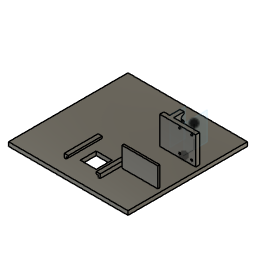
tapa mecatronica v7 (Autodesk Fusion 360 design; units mm, degrees)
Autodesk Fusion 360 part; units mm, degrees
sketch "Boceto1" plane through (0, 0, 0) normal (0, 0, 1) x (1, 0, 0)
  line L0 (-150, -150) -> (150, -150)
  line L1 (150, -150) -> (150, 150)
  line L2 (150, 150) -> (-150, 150)
  line L3 (-150, 150) -> (-150, -150)
  dimension "d1" = 300
  dimension "d2" = 300
  constraint horizontal L0
  constraint vertical L1
  constraint horizontal L2
  constraint vertical L3
  measures "d1" distance of L0.start L0.end
  measures "d2" distance of L0.start L2.end
extrude "Extruir1" add sketch "Boceto1" along normal blind 10
sketch "Boceto2" plane through (0, 0, 10) normal (0, 0, 1) x (-1, 0, 0)
  line L0 (150, -150) -> (150, 150)
  line L1 (150, 150) -> (-150, 150)
  line L2 (-150, 150) -> (-150, -150)
  line L3 (-150, -150) -> (150, -150)
  line L4 (20, 100) -> (-20, 100)
  line L5 (-20, 100) -> (-20, 60)
  line L6 (-20, 60) -> (20, 60)
  line L7 (20, 60) -> (20, 100)
  dimension "d5" = 40
  dimension "d6" = 40
  constraint horizontal L4
  constraint vertical L5
  constraint horizontal L6
  constraint vertical L7
  measures "d5" distance of L5.end L6.end
  measures "d6" distance of L4.start L6.end
shell "Vaciado1" thickness 10 removed faces 1 at (-50, 50, 10)
extrude "Extruir2" cut sketch "Boceto2" against normal blind 10 contours L4 L5 L6 L7
sketch "Boceto3" plane through (0, 0, 10) normal (0, 0, 1) x (-1, 0, 0)
  line L0 (-20, 100) -> (20, 100)
  line L1 (20, 100) -> (20, 60)
  line L2 (20, 60) -> (-20, 60)
  line L3 (-20, 60) -> (-20, 100)
  line L4 (150, -150) -> (150, 150)
  line L5 (150, 150) -> (-150, 150)
  line L6 (-150, 150) -> (-150, -150)
  line L7 (-150, -150) -> (150, -150)
  line L8 (-50, 60) -> (-140, 60)
  line L9 (-140, 60) -> (-140, 65)
  line L10 (-140, 65) -> (-50, 65)
  line L11 (-50, 65) -> (-50, 60)
  constraint horizontal L8
  constraint vertical L9
  constraint horizontal L10
  constraint vertical L11
extrude "Extruir3" add sketch "Boceto3" along normal blind 50 contours L8 L9 L10 L11
sketch "Boceto4" plane through (0, 0, 10) normal (0, 0, 1) x (-1, 0, 0)
  line L0 (-50, 65) -> (-50, 60)
  line L1 (-50, 60) -> (-140, 60)
  line L2 (-140, 60) -> (-140, 65)
  line L3 (-140, 65) -> (-50, 65)
  line L4 (-20, 100) -> (20, 100)
  line L5 (20, 100) -> (20, 60)
  line L6 (20, 60) -> (-20, 60)
  line L7 (-20, 60) -> (-20, 100)
  line L8 (150, -150) -> (150, 150)
  line L9 (150, 150) -> (-150, 150)
  line L10 (-150, 150) -> (-150, -150)
  line L11 (-150, -150) -> (150, -150)
  line L12 (45, 30) -> (40, 30)
  line L13 (40, 30) -> (40, 115)
  line L14 (40, 115) -> (45, 115)
  line L15 (45, 115) -> (45, 30)
  line L16 (35, 30) -> (30, 30)
  line L17 (30, 30) -> (30, 115)
  line L18 (30, 115) -> (35, 115)
  line L19 (35, 115) -> (35, 30)
  line L20 (-30, 30) -> (-35, 30)
  line L21 (-35, 30) -> (-35, 115)
  line L22 (-35, 115) -> (-30, 115)
  line L23 (-30, 115) -> (-30, 30)
  line L24 (-40, 30) -> (-45, 30)
  line L25 (-45, 30) -> (-45, 115)
  line L26 (-45, 115) -> (-40, 115)
  line L27 (-40, 115) -> (-40, 30)
  constraint horizontal L12
  constraint vertical L13
  constraint horizontal L14
  constraint vertical L15
  constraint horizontal L16
  constraint vertical L17
  constraint horizontal L18
  constraint vertical L19
  constraint horizontal L20
  constraint vertical L21
  constraint horizontal L22
  constraint vertical L23
  constraint horizontal L24
  constraint vertical L25
  constraint horizontal L26
  constraint vertical L27
extrude "Extruir4" add sketch "Boceto4" along normal blind 10 contours L12 L13 L14 L15 | L16 L17 L18 L19 | L20 L21 L22 L23 | L24 L25 L26 L27
sketch "Boceto5" plane through (-40, 0, 0) normal (1, 0, 0) x (0, 1, 0)
  line L0 (-115, 10) -> (-30, 10)
  line L1 (-30, 10) -> (-30, 20)
  line L2 (-30, 20) -> (-115, 20)
  line L3 (-115, 20) -> (-115, 10)
  line L4 (-30, 20) -> (-115, 20)
  line L5 (-115, 20) -> (-115, 15)
  line L6 (-115, 15) -> (-30, 15)
  line L7 (-30, 15) -> (-30, 20)
  constraint horizontal L4
  constraint vertical L5
  constraint horizontal L6
  constraint vertical L7
  constraint midpoint L3 L5.end
  constraint coincident L1.end L2.start
extrude "Extruir5" add sketch "Boceto5" along normal blind 5 contours L1 L2 L3 L4 L5 L6 L7
sketch "Boceto6" plane through (35, 0, 0) normal (1, 0, 0) x (0, 1, 0)
  line L0 (-115, 10) -> (-30, 10)
  line L1 (-30, 10) -> (-30, 20)
  line L2 (-30, 20) -> (-115, 20)
  line L3 (-115, 20) -> (-115, 10)
  line L4 (-30, 20) -> (-115, 20)
  line L5 (-115, 20) -> (-115, 15)
  line L6 (-115, 15) -> (-30, 15)
  line L7 (-30, 15) -> (-30, 20)
  constraint horizontal L4
  constraint vertical L5
  constraint horizontal L6
  constraint vertical L7
  constraint midpoint L3 L5.end
  constraint coincident L1.end L2.start
extrude "Extruir6" add sketch "Boceto6" along normal blind 5 contours L1 L2 L3 L4 L5 L6 L7
sketch "Boceto7" plane through (0, 0, 20) normal (0, 0, 1) x (-1, 0, 0)
  line L0 (-30, 115) -> (-45, 115)
  line L1 (-45, 115) -> (-45, 30)
  line L2 (-45, 30) -> (-30, 30)
  line L3 (-30, 30) -> (-30, 115)
  line L4 (-30, 30) -> (-35, 30)
  line L5 (-35, 30) -> (-35, 115)
  line L6 (-35, 115) -> (-30, 115)
  line L7 (-30, 115) -> (-30, 30)
  constraint horizontal L4
  constraint vertical L5
  constraint horizontal L6
  constraint vertical L7
  constraint coincident L0 L5.end
  constraint coincident L2.end L3.start
extrude "Extruir7" cut sketch "Boceto7" against normal blind 10 contours L0 L2 L3 L4 L5 L6 L7
sketch "Boceto8" plane through (0, 0, 20) normal (0, 0, 1) x (-1, 0, 0)
  line L0 (45, 115) -> (30, 115)
  line L1 (30, 115) -> (30, 30)
  line L2 (30, 30) -> (45, 30)
  line L3 (45, 30) -> (45, 115)
  line L4 (30, 30) -> (35, 30)
  line L5 (35, 30) -> (35, 115)
  line L6 (35, 115) -> (30, 115)
  line L7 (30, 115) -> (30, 30)
  constraint horizontal L4
  constraint vertical L5
  constraint horizontal L6
  constraint vertical L7
  constraint coincident L0 L5.end
  constraint coincident L1.end L2.start
extrude "Extruir8" cut sketch "Boceto8" against normal blind 10 contours L0 L1 L2 L4 L5 L6 L7
sketch "Boceto9" plane through (0, 0, 10) normal (0, 0, 1) x (-1, 0, 0)
  line L0 (-40, 115) -> (-40, 30)
  line L1 (-40, 30) -> (-45, 30)
  line L2 (-45, 30) -> (-45, 115)
  line L3 (-45, 115) -> (-40, 115)
  line L4 (45, 115) -> (45, 30)
  line L5 (45, 30) -> (40, 30)
  line L6 (40, 30) -> (40, 115)
  line L7 (40, 115) -> (45, 115)
  line L8 (-50, 65) -> (-50, 60)
  line L9 (-50, 60) -> (-140, 60)
  line L10 (-140, 60) -> (-140, 65)
  line L11 (-140, 65) -> (-50, 65)
  line L12 (-20, 100) -> (20, 100)
  line L13 (20, 100) -> (20, 60)
  line L14 (20, 60) -> (-20, 60)
  line L15 (-20, 60) -> (-20, 100)
  line L16 (150, -150) -> (150, 150)
  line L17 (150, 150) -> (-150, 150)
  line L18 (-150, 150) -> (-150, -150)
  line L19 (-150, -150) -> (150, -150)
  line L20 (-53.6432, 60) -> (-53.6432, -53) construction
  line L21 (-50, -30) -> (-140, -30)
  line L22 (-140, -30) -> (-140, -40)
  line L23 (-140, -40) -> (-50, -40)
  line L24 (-50, -40) -> (-50, -30)
  dimension "d22" = 113
  constraint coincident L9 L20.start
  constraint perpendicular L9 L20
  constraint horizontal L21
  constraint vertical L22
  constraint horizontal L23
  constraint vertical L24
  measures "d22" distance of L20.start L20.end
extrude "Extruir9" add sketch "Boceto9" along normal blind 70 contours L21 L22 L23 L24
sketch "Boceto10" plane through (0, 0, 10) normal (0, 0, 1) x (-1, 0, 0)
  line L0 (-50, -40) -> (-140, -40)
  line L1 (-140, -40) -> (-140, -30)
  line L2 (-140, -30) -> (-50, -30)
  line L3 (-50, -30) -> (-50, -40)
  line L4 (-40, 115) -> (-40, 30)
  line L5 (-40, 30) -> (-45, 30)
  line L6 (-45, 30) -> (-45, 115)
  line L7 (-45, 115) -> (-40, 115)
  line L8 (45, 115) -> (45, 30)
  line L9 (45, 30) -> (40, 30)
  line L10 (40, 30) -> (40, 115)
  line L11 (40, 115) -> (45, 115)
  line L12 (-50, 65) -> (-50, 60)
  line L13 (-50, 60) -> (-140, 60)
  line L14 (-140, 60) -> (-140, 65)
  line L15 (-140, 65) -> (-50, 65)
  line L16 (-20, 100) -> (20, 100)
  line L17 (20, 100) -> (20, 60)
  line L18 (20, 60) -> (-20, 60)
  line L19 (-20, 60) -> (-20, 100)
  line L20 (150, -150) -> (150, 150)
  line L21 (150, 150) -> (-150, 150)
  line L22 (-150, 150) -> (-150, -150)
  line L23 (-150, -150) -> (150, -150)
  line L24 (-100, -40) -> (-133.3526, -40)
  line L25 (-133.3526, -40) -> (-133.3526, -99.3533)
  line L26 (-133.3526, -99.3533) -> (-100, -99.3533)
  line L27 (-100, -99.3533) -> (-100, -40)
  constraint horizontal L24
  constraint vertical L25
  constraint horizontal L26
  constraint vertical L27
  constraint coincident L0 L24.start
extrude "Extruir10" add sketch "Boceto10" along normal blind 70 contours L0 L24 L25 L26 L27
sketch "Boceto11" plane through (100, 0, 0) normal (-1, 0, 0) x (0, -1, 0)
  line L0 (-99.3533, 10) -> (-40, 10)
  line L1 (-40, 10) -> (-40, 80)
  line L2 (-40, 80) -> (-99.3533, 80)
  line L3 (-99.3533, 80) -> (-99.3533, 10)
  line L4 (-40, 10) -> (-65.989, 10) construction
  line L5 (-65.989, 10) -> (-65.989, 67.376) construction
  dimension "d27" = 25.989
  dimension "d28" = 57.376
  constraint coincident L0.end L1.start
  constraint perpendicular L1 L4
  constraint perpendicular L0 L5
  measures "d27" distance of L0.end L4.end
  measures "d28" distance of L4.end L5.end
sketch "Boceto12" plane through (100, 0, 0) normal (-1, 0, 0) x (0, -1, 0)
  circle A0 centre (-66.0255, 67.4058) radius 7.5
  dimension "d30" = 15
  measures "d30" diameter of A0
extrude "Extruir11" cut sketch "Boceto12" against normal blind 10
sketch "Boceto13" plane through (100, 0, 0) normal (-1, 0, 0) x (0, -1, 0)
sketch "Boceto14" plane through (0, 0, 10) normal (0, 0, 1) x (-1, 0, 0)
  line L0 (150, -150) -> (150, 150)
  line L1 (150, 150) -> (-150, 150)
  line L2 (-150, 150) -> (-150, -150)
  line L3 (-150, -150) -> (150, -150)
  line L4 (-20, 100) -> (20, 100)
  line L5 (20, 100) -> (20, 60)
  line L6 (20, 60) -> (-20, 60)
  line L7 (-20, 60) -> (-20, 100)
  line L8 (-50, 65) -> (-50, 60)
  line L9 (-50, 60) -> (-140, 60)
  line L10 (-140, 60) -> (-140, 65)
  line L11 (-140, 65) -> (-50, 65)
  line L12 (45, 115) -> (45, 30)
  line L13 (45, 30) -> (40, 30)
  line L14 (40, 30) -> (40, 115)
  line L15 (40, 115) -> (45, 115)
  line L16 (-40, 115) -> (-40, 30)
  line L17 (-40, 30) -> (-45, 30)
  line L18 (-45, 30) -> (-45, 115)
  line L19 (-45, 115) -> (-40, 115)
  line L20 (-100, -40) -> (-100, -99.3533)
  line L21 (-100, -99.3533) -> (-133.3526, -99.3533)
  line L22 (-133.3526, -99.3533) -> (-133.3526, -40)
  line L23 (-133.3526, -40) -> (-140, -40)
  line L24 (-140, -40) -> (-140, -30)
  line L25 (-140, -30) -> (-50, -30)
  line L26 (-50, -30) -> (-50, -40)
  line L27 (-50, -40) -> (-100, -40)
  line L28 (-65, -40) -> (-75, -40)
  line L29 (-75, -40) -> (-75, -79)
  line L30 (-75, -79) -> (-65, -79)
  line L31 (-65, -79) -> (-65, -40)
  constraint horizontal L28
  constraint vertical L29
  constraint horizontal L30
  constraint vertical L31
  constraint coincident L27 L28.start
extrude "Extruir12" add sketch "Boceto14" along normal blind 70 contours L27 L28 L29 L30 L31
sketch "Boceto15" plane through (100, 0, 0) normal (-1, 0, 0) x (0, -1, 0)
  circle A0 centre (-66, 67.4) radius 7.5
  dimension "d35" = 15
  measures "d35" diameter of A0
extrude "Extruir13" cut sketch "Boceto15" along normal blind 100
sketch "Boceto16" plane through (0, 0, 80) normal (0, 0, 1) x (-1, 0, 0)
  line L0 (-50, -40) -> (-50, -30)
  line L1 (-50, -30) -> (-140, -30)
  line L2 (-140, -30) -> (-140, -40)
  line L3 (-140, -40) -> (-133.3526, -40)
  line L4 (-133.3526, -40) -> (-133.3526, -99.3533)
  line L5 (-133.3526, -99.3533) -> (-100, -99.3533)
  line L6 (-100, -99.3533) -> (-100, -40)
  line L7 (-100, -40) -> (-75, -40)
  line L8 (-75, -40) -> (-75, -79)
  line L9 (-75, -79) -> (-65, -79)
  line L10 (-65, -79) -> (-65, -40)
  line L11 (-65, -40) -> (-50, -40)
  line L12 (-100, -99.3533) -> (-133.3526, -99.3533)
  line L13 (-133.3526, -99.3533) -> (-133.3526, -40)
  line L14 (-133.3526, -40) -> (-100, -40)
  line L15 (-100, -40) -> (-100, -99.3533)
  constraint horizontal L12
  constraint vertical L13
  constraint horizontal L14
  constraint vertical L15
  constraint coincident L3.end L4.start
  constraint coincident L5.end L6.start
extrude "Extruir14" cut sketch "Boceto16" against normal blind 70 contours L4 L5 L6 L12 L13 L14 L15
sketch "Boceto17" plane through (65, 0, 0) normal (-1, 0, 0) x (0, -1, 0)
  circle A0 centre (-66, 67.4) radius 7.5
  line L0 (-79, 10) -> (-40, 10)
  line L1 (-40, 10) -> (-40, 80)
  line L2 (-40, 80) -> (-79, 80)
  line L3 (-79, 80) -> (-79, 10)
sketch "Boceto18" plane through (65, 0, 0) normal (-1, 0, 0) x (0, -1, 0)
  line L0 (-66, 10) -> (-79, 10)
  line L1 (-79, 10) -> (-79, 80)
  line L2 (-79, 80) -> (-66, 80)
  line L3 (-66, 80) -> (-66, 10)
  constraint horizontal L0
  constraint vertical L1
  constraint horizontal L2
  constraint vertical L3
extrude "Extruir15" cut sketch "Boceto18" against normal blind 10
sketch "Boceto19" plane through (0, 40, 0) normal (0, 1, 0) x (-1, 0, 0)
  line L0 (-75, 80) -> (-140, 80)
  line L1 (-140, 80) -> (-140, 10)
  line L2 (-140, 10) -> (-75, 10)
  line L3 (-75, 10) -> (-75, 80)
  circle A0 centre (-130, 75) radius 2.5
  circle A1 centre (-100, 75) radius 2.5
  circle A2 centre (-130, 20) radius 2.5
  circle A3 centre (-100, 20) radius 2.5
  dimension "d42" = 5
  dimension "d43" = 5
  dimension "d44" = 5
  dimension "d45" = 5
  measures "d42" diameter of A0
  measures "d43" diameter of A1
  measures "d44" diameter of A2
  measures "d45" diameter of A3
extrude "Extruir16" cut sketch "Boceto19" against normal blind 10 contours A0 | A1 | A2 | A3
